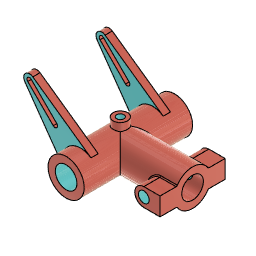
Exercise-26 v0 (Autodesk Fusion 360 design; units mm, degrees)
Autodesk Fusion 360 part; units mm, degrees
note: some values were not read from the file. Set by a fixed rule: which sketch regions a step uses.
sketch "Sketch1" plane through (0, 0, 0) normal (0, 1, 0) x (1, 0, 0)
  circle A0 centre (0, 0) radius 15
  circle A1 centre (0, 0) radius 25
  line L0 (0, 0) -> (-70.7107, -70.7107) construction
  line L1 (0, 0) -> (100, 0) construction
  circle A2 centre (-70.7107, -70.7107) radius 8
  line L2 (-77.2469, -66.0978) -> (-20.4256, 14.4152)
  line L3 (-66.0978, -77.2469) -> (14.4152, -20.4256)
  line L4 (-68.2358, -73.1856) -> (-32.8805, -37.8302)
  arc A3 (-32.8805, -37.8302) -> (-37.8302, -32.8805) centre (-35.3553, -35.3553) ccw
  line L5 (-37.8302, -32.8805) -> (-73.1856, -68.2358)
  arc A4 (-73.1856, -68.2358) -> (-68.2358, -73.1856) centre (-70.7107, -70.7107) ccw
  line L6 (-70.7107, -70.7107) -> (-35.3553, -35.3553) construction
  dimension "d1" = 30
  dimension "d2" = 50
  dimension "d3" = 135
  dimension "d4" = 100
  dimension "d5" = 16
  dimension "d6" = 50
  dimension "d7" = 7
  constraint coincident A0.centre A1.centre
  constraint concentric A0 A1
  constraint horizontal L1
  constraint coincident L0.end A2.centre
  constraint coincident A2 L2.start
  constraint coincident A1 L2.end
  constraint tangent A1 L2
  constraint coincident A2 L3.start
  constraint coincident A1 L3.end
  constraint tangent A1 L3
  constraint tangent A2 L3
  constraint tangent A2 L2
  constraint tangent L4 A3
  constraint tangent A3 L5
  constraint parallel L4 L5
  constraint tangent L5 A4
  constraint tangent L4 A4
  constraint parallel L0 L6
  measures "d1" diameter of A0
  measures "d2" diameter of A1
  measures "d3" angle of L0 L1
  measures "d4" distance of A0.centre L0.end
  measures "d5" diameter of A2
  measures "d6" distance of L0.end A3.centre
  measures "d7" diameter of A3
extrude "Extrude1" add sketch "Sketch1" along normal mid plane 150 contours A1
extrude "Extrude2" add sketch "Sketch1" along normal blind 10 from surface at 45 contours A1 A2 L2 L3 L4 A3 L5 | A2 L4 L5 A4 picked at (-76.3018, -67.4269)
mirror "Mirror1" about plane through (0, 0, 0) normal (0, 1, 0) of "Extrude2"
sketch "Sketch2" plane through (0, 0, 0) normal (1, 0, 0) x (0, 1, 0)
  line L0 (-45, 66.0978) -> (-45, 25)
  line L1 (-55, 25) -> (-55, 66.0978)
  line L2 (-45, 66.0978) -> (-45, 78.7107)
  line L3 (-55, 66.0978) -> (-55, 78.7107)
  line L4 (-75, 0) -> (-75, -25)
  line L5 (-75, 25) -> (-75, 0)
  line L6 (75, 0) -> (75, 25)
  line L7 (75, -25) -> (75, 0)
  line L8 (45, 66.0978) -> (45, 25)
  line L9 (55, 25) -> (55, 66.0978)
  line L10 (45, 66.0978) -> (45, 78.7107)
  line L11 (55, 66.0978) -> (55, 78.7107)
  line L12 (-55, 78.7107) -> (-45, 78.7107)
  line L13 (-75, -25) -> (75, -25)
  line L14 (-75, 25) -> (-55, 25)
  line L15 (-45, 25) -> (45, 25)
  line L16 (55, 25) -> (75, 25)
  line L17 (45, 78.7107) -> (55, 78.7107)
  circle A0 centre (0, 0) radius 25
  circle A1 centre (0, 0) radius 15
  line L18 (-45, 12.5) -> (-45, -12.5)
  line L19 (-45, -12.5) -> (-21.6506, -12.5)
  line L20 (-45, 12.5) -> (-21.6506, 12.5)
  dimension "d15" = 50
  dimension "d16" = 30
  dimension "d17" = 25
  dimension "d18" = 12.5
  constraint coincident A0.centre A1.centre
  constraint concentric A0 A1
  constraint vertical L18
  constraint coincident A0 L19.end
  constraint perpendicular L18 L19
  constraint coincident A0 L20.end
  constraint perpendicular L18 L20
  measures "d15" diameter of A0
  measures "d16" diameter of A1
  measures "d17" distance of L18.start L18.end
  measures "d18" vertical distance of A0.centre L18.start
extrude "Extrude3" add sketch "Sketch2" along normal blind 100 contours A0
extrude "Extrude4" cut sketch "Sketch1" along normal mid plane 150 contours A0
extrude "Extrude5" add sketch "Sketch2" against normal blind 35 from surface at 100 contours A0 L18 L19 L20
mirror "Mirror2" about plane through (0, 0, 0) normal (0, 1, 0) of "Extrude5"
fillet "Fillet1" radius 12.5 4 edges at (65, -33.3253, 12.5) (65, -33.3253, -12.5) (65, 33.3253, 12.5) (65, 33.3253, -12.5)
fillet "Fillet2" radius 2 8 edges at (88.75, 21.6506, 12.5) (68.6701, 23.382, 8.8478) (68.6701, 23.382, -8.8478) (88.75, 21.6506, -12.5) (88.75, -21.6506, -12.5) (68.6701, -23.382, -8.8478) (68.6701, -23.382, 8.8478) (88.75, -21.6506, 12.5)
hole "Hole1" at (77.5, -45, 0) direction (0, 1, 0) diameter 15 end through all
ref_plane "WorkPlane1" through (0, 0, 35) normal (0, 0, 1) x (1, 0, 0)
sketch "Sketch3" plane through (0, 0, 35) normal (0, 0, 1) x (1, 0, 0)
  circle A0 centre (0, 0) radius 10
  circle A1 centre (0, 0) radius 5
  dimension "d35" = 20
  dimension "d36" = 10
  constraint coincident A0.centre A1.centre
  measures "d35" diameter of A0
  measures "d36" diameter of A1
extrude "Extrude6" add sketch "Sketch3" against normal blind 15
extrude "Extrude7" cut sketch "Sketch3" against normal blind 30 contours A1
